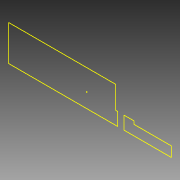
# Autodesk Inventor part: NegTerm
Saved by Autodesk Inventor 2014 (Build 180170000, 170)
## iProperties
Created: 2014-11-22
Part Number: NegTerm
Material: Nickel-Copper Alloy 400
Document SubType Name: Modeling
Designer: DV
Mass: 0.00863769 g
Surface Area: 0.212956 cm^2
Volume: 0.000978221 cm^3
Density: 8.83 g/cm^3
Appearance: Chrome - Polished
Author: DV
Autodesk Inventor part; units mm, degrees
ref_plane "YZ Plane" through (0, 0, 0) normal (1, 0, 0) x (0, 1, 0)
ref_plane "XZ Plane" through (0, 0, 0) normal (0, 1, 0) x (-1, 0, 0)
ref_plane "XY Plane" through (0, 0, 0) normal (0, 0, 1) x (1, 0, 0)
sketch "Sketch2" plane through (0, 0, 0) normal (0, 0, 1) x (1, 0, 0)
  line L0 (-3.2347, 1.0674) -> (-3.2347, -0.8326) projected
  line L1 (-3.2347, -0.8326) -> (1.2942, -0.8326) projected
  line L2 (3.5212, -0.8326) -> (3.5212, -0.2505) projected
  line L3 (1.2017, 1.0674) -> (-3.2347, 1.0674) projected
  line L4 (3.5212, 1.0674) -> (-3.2347, 1.0674)
  line L5 (-3.2347, 1.0674) -> (-3.2347, -0.8326)
  line L6 (-3.2347, 0.1174) -> (3.5212, 0.1174) construction
  line L7 (1.9688, -0.1158) -> (1.5482, -0.1158) construction
  line L8 (3.5212, -0.2505) -> (1.9688, -0.2505) construction
  line L9 (1.5482, -0.8326) -> (1.5482, -0.1158) projected
  line L10 (1.5482, -0.8326) -> (3.5212, -0.8326) projected
  line L11 (3.5212, -0.8326) -> (3.5212, -0.2505) projected
  line L12 (3.5212, -0.2505) -> (1.9688, -0.2505) projected
  line L13 (1.9688, -0.2505) -> (1.9688, -0.1158) projected
  line L14 (1.9688, -0.1158) -> (1.5482, -0.1158) projected
  line L15 (1.9688, 0.3505) -> (1.5482, 0.3505) construction
  line L16 (3.5212, 0.4853) -> (1.9688, 0.4853) construction
  line L17 (3.5212, 0.4853) -> (1.9688, 0.4853)
  line L18 (1.9688, 0.3505) -> (1.1168, 0.3505)
  line L19 (1.1168, 0.3505) -> (1.1168, -0.8326)
  line L20 (1.9688, 0.4853) -> (1.9688, 0.3505)
  line L21 (3.5212, -0.8326) -> (3.5212, 0.1174)
  line L22 (3.5212, 0.4853) -> (3.5212, 1.0674)
  line L23 (-3.2347, -0.8326) -> (1.1168, -0.8326)
  line L24 (1.5482, -0.8326) -> (3.5212, -0.8326)
  circle A0 centre (-2.3788, 0.1174) radius 0.122 projected
  point P0 (0, 0)
  constraints: 23 end point, 5 parallel, 5 perpendicular, 4 symmetric about line, 2 horizontal, 1 collinear, 1 midpoint, 1 point on line
extrude "Extrusion1" add sketch "Sketch2" along normal blind 0.1 contours L3 L4 L22 L17 L20 L18 L19 L1 L0
body "Solid1"
